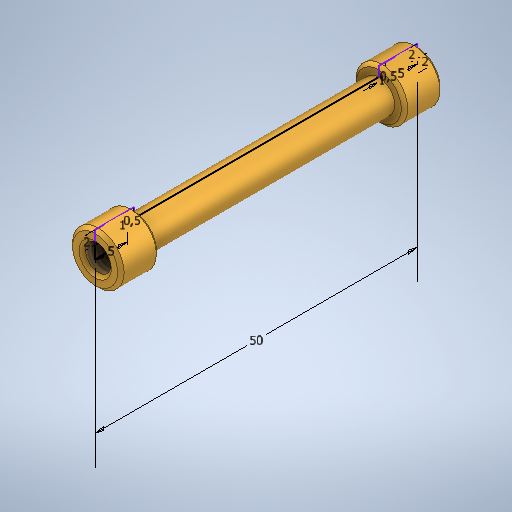
# Autodesk Inventor part: Heater
Saved by Autodesk Inventor 2025.2 (Build 292293000, 293)
## iProperties
Created: 2026-06-11
Part Number: Heater
Material: Generic
Document SubType Name: Modeling
Designer: Simon
Density: 1 g/cm^3
Appearance: Brass - Satin
Author: Simon
Autodesk Inventor part; units mm, degrees
ref_plane "YZ Plane" through (0, 0, 0) normal (1, 0, 0) x (0, 1, 0)
ref_plane "XZ Plane" through (0, 0, 0) normal (0, 1, 0) x (-1, 0, 0)
ref_plane "XY Plane" through (0, 0, 0) normal (0, 0, 1) x (1, 0, 0)
sketch "Sketch1" plane through (0, 0, 0) normal (1, 0, 0) x (0, 1, 0)
  line L0 (0, 0) -> (0, -50)
  line L1 (0, -50) -> (2, -50)
  line L2 (2, -50) -> (2, 0)
  line L3 (2, 0) -> (0, 0)
  line L4 (2, 0) -> (2, -5)
  line L5 (2, -50) -> (2, -45)
  line L6 (2, -50) -> (4, -50)
  line L7 (4, -50) -> (4, -45)
  line L8 (4, -45) -> (2, -45)
  line L9 (2, 0) -> (4, 0)
  line L10 (4, 0) -> (4, -5)
  line L11 (4, -5) -> (2, -5)
  line L12 (2, -45) -> (1.5, -45)
  line L13 (1.5, -45) -> (1.5, -5)
  line L14 (1.5, -5) -> (2, -5)
  line L15 (4, -5) -> (4, -6)
  line L16 (4, -6) -> (1.5, -6)
  line L17 (4, -45) -> (4, -44)
  line L18 (4, -44) -> (1.5, -44)
  line L19 (2, -6) -> (2.5, -6)
  line L20 (2.5, -6) -> (2.5, -44)
  point P0 (2, -44)
  dimension "d0" = 50
  dimension "d1" = 2
  dimension "d2" = 5
  dimension "d3" = 5
  dimension "d5" = 2
  dimension "d6" = 2
  dimension "d7" = 0.5
  dimension "d8" = 1
  dimension "d9" = 1
  dimension "d21" = 0.5
  constraints: 42 end point, 11 point on line, 10 perpendicular, 2 vertical, 1 horizontal, 1 parallel
  measures "d0" distance of L0.start L0.end
  measures "d1" distance of L0.end L1.end
  measures "d2" distance of L2.end L4.end
  measures "d3" distance of L1.end L5.end
  measures "d5" distance of L1.end L6.end
  measures "d6" distance of L2.end L9.end
  measures "d7" distance of L5.end L12.end
  measures "d8" distance of L10.end L15.end
  measures "d9" distance of L7.end L17.end
  measures "d21" distance of L19.start L19.end
revolve "Revolution1" add sketch "Sketch1" angle 360 about axis through (0, 0, 0) along (0, 0, -1) contours L9 L10 L11 L2 | L2 L8 L7 L6 | L11 L15 L16 L2 | L2 L16 L13 L14 | L12 L13 L18 L2 | L2 L18 L17 L8 | L16 L20 L18 L2 | L2 L18 L13 L16
thread "Thread1" size "M4x0.7" class "6H" standard "ANSI Metric M Profile" full length
thread "Thread2" size "M4x0.7" class "6H" standard "ANSI Metric M Profile" full length
chamfer "Chamfer1" distance 0.5 angle 45 2 edges at (0, -2, 0) (0, -2, -50)
chamfer "Chamfer2" distance 0.5 angle 45 4 edges at (0, -4, -50) (0, -4, -44) (0, -4, -6) (0, -4, 0)
body "Solid1"
